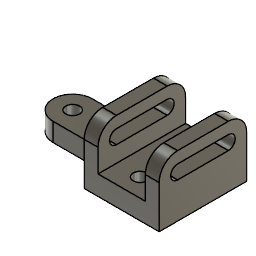
ISO 4 (Autodesk Fusion 360 design; units mm, degrees)
part number: 2026-02-06-11-06-08-759
Autodesk Fusion 360 part; units mm, degrees
sketch "Sketch1" plane through (0, 0, 0) normal (0, 0, 1) x (1, 0, 0)
  circle A0 centre (-48, 0) radius 6
  line L0 (-48, -17) -> (0, -17)
  line L1 (-48, 17) -> (0, 17)
  line L2 (0, 17) -> (0, -17)
  arc A1 (-48, 17) -> (-48, -17) centre (-48, 0) ccw
  dimension "d1" = 48
  dimension "d2" = 12
  dimension "d3" = 34
  dimension "d5" = 48
  constraint concentric A0 A1
  constraint horizontal L0
  constraint horizontal L1
  constraint perpendicular L0 L2
  measures "d1" distance of origin A0.centre
  measures "d2" diameter of A0
  measures "d3" diameter of A1
  measures "d5" distance of L1.start L1.end
extrude "Extrude1" add sketch "Sketch1" along normal mid plane 16
sketch "Sketch2" plane through (0, 0, 0) normal (0, 1, 0) x (1, 0, 0)
  line L0 (0, 8) -> (65, 8)
  line L1 (0, 8) -> (0, -45)
  line L2 (0, -45) -> (12, -45)
  line L3 (12, -45) -> (12, -9)
  line L4 (12, -9) -> (53, -9)
  line L5 (65, 8) -> (65, -45)
  line L6 (65, -45) -> (53, -45)
  line L7 (53, -45) -> (53, -9)
  dimension "d8" = 65
  dimension "d9" = 53
  dimension "d10" = 12
  dimension "d11" = 41
  dimension "d12" = 53
  dimension "d13" = 12
  constraint horizontal L0
  constraint perpendicular L0 L1
  constraint perpendicular L1 L2
  constraint perpendicular L2 L3
  constraint perpendicular L3 L4
  constraint perpendicular L0 L5
  constraint perpendicular L5 L6
  measures "d8" distance of L0.start L0.end
  measures "d9" distance of L0.start L1.end
  measures "d10" distance of L1.end L2.end
  measures "d11" distance of L3.end L4.end
  measures "d12" distance of L0.end L5.end
  measures "d13" distance of L5.end L6.end
extrude "Extrude2" add sketch "Sketch2" along normal mid plane 76
fillet "Fillet1" radius 16 4 edges at (6, 38, 45) (6, -38, 45) (59, -38, 45) (59, 38, 45)
sketch "Sketch3" plane through (0, 0, 0) normal (-1, 0, 0) x (0, -1, 0)
  arc A0 (38, 29) -> (22, 45) centre (22, 29) ccw
  line L0 (22, 45) -> (-22, 45)
  arc A1 (-22, 45) -> (-38, 29) centre (-22, 29) ccw
  line L1 (-38, 29) -> (-38, -8)
  line L2 (-38, -8) -> (-17, -8)
  line L3 (-17, -8) -> (-17, 8)
  line L4 (-17, 8) -> (17, 8)
  line L5 (17, 8) -> (17, -8)
  line L6 (17, -8) -> (38, -8)
  line L7 (38, -8) -> (38, 29)
  line L8 (-22, 23) -> (22, 23)
  arc A2 (22, 23) -> (22, 35) centre (22, 29) ccw
  line L9 (22, 35) -> (-22, 35)
  arc A3 (-22, 35) -> (-22, 23) centre (-22, 29) ccw
  line L10 (-22, 29) -> (22, 29) construction
  dimension "d18" = 44
  dimension "d19" = 6
  dimension "d21" = 21
  constraint tangent L8 A2
  constraint tangent A2 L9
  constraint parallel L8 L9
  constraint tangent L9 A3
  constraint tangent L8 A3
  constraint horizontal L10
  constraint concentric A1 A3
  measures "d18" distance of A1.centre A0.centre
  measures "d19" radius of A3
  measures "d21" vertical distance of L3.end A1.centre
extrude "Extrude3" cut sketch "Sketch3" against normal blind 65 contours L8 A2 L9 A3
sketch "Sketch4" plane through (0, 0, 9) normal (0, 0, 1) x (-1, 0, 0)
  line L0 (-53, 38) -> (-53, -38)
  line L1 (-53, -38) -> (-12, -38)
  line L2 (-12, -38) -> (-12, 38)
  line L3 (-12, 38) -> (-53, 38)
  point P0 (-32.5, -22)
  point P1 (-32.5, 22)
  dimension "d24" = 44
  dimension "d25" = 16
  dimension "d26" = 20.5
  constraint vertical P0 P1
  measures "d24" distance of P0 P1
  measures "d25" distance of L1 P0
  measures "d26" distance of L2 P0
hole "Hole1" at (32.5, 22, 9) at (32.5, -22, 9) direction (0, 0, -1) diameter 12 depth 65 tip angle 118
